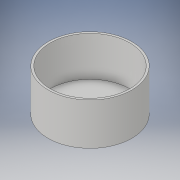
# Autodesk Inventor part: base redonda
Saved by Autodesk Inventor 2019 (Build 230136000, 136)
## iProperties
Created: 2019-10-18
Part Number: base redonda
Material: Genérico
Document SubType Name: Modeling
Designer: Josue
Density: 1 g/cm^3
Appearance: Valor por defecto
Author: Josue
Autodesk Inventor part; units mm, degrees
ref_plane "YZ Plane" through (0, 0, 0) normal (1, 0, 0) x (0, 1, 0)
ref_plane "XZ Plane" through (0, 0, 0) normal (0, 1, 0) x (-1, 0, 0)
ref_plane "XY Plane" through (0, 0, 0) normal (0, 0, 1) x (1, 0, 0)
sketch "Boceto1" plane through (0, 0, 0) normal (0, 1, 0) x (-1, 0, 0)
  circle A0 centre (0, 0) radius 100
  dimension "d0" = 200
  constraints: 1 centre point, 1 coincident
  measures "d0" diameter of A0
extrude "Extrusión1" add sketch "Boceto1" along normal mid plane 100
shell "Vaciado1" thickness 5 removed faces 1 at (-44.3571, 50, 16.5389)
sketch "Boceto2" plane through (0, -50, 0) normal (0, -1, 0) x (1, 0, 0)
  point P0 (0, 0)
  point P1 (0.1915, 0)
hole "Agujero1" at (0.1915, -50, 0) direction (0, 1, 0) diameter 40.241 end through all
